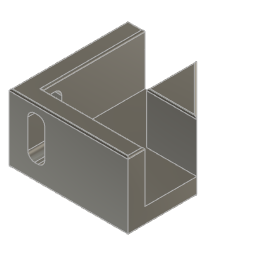
1515 (Autodesk Fusion 360 design; units mm, degrees)
Autodesk Fusion 360 part; units mm, degrees
sketch "Sketch1" plane through (0, 0, 0) normal (0, 0, 1) x (1, 0, 0)
  line L0 (0, 0) -> (35, 0)
  line L1 (35, 0) -> (35, 35)
  line L2 (35, 35) -> (0, 35)
  line L3 (0, 35) -> (0, 0)
  dimension "d1" = 35
  dimension "d2" = 35
  constraint horizontal L0
  constraint vertical L1
  constraint horizontal L2
  constraint vertical L3
  constraint coincident L0.start L3.end
  measures "d1" distance of L0.start L0.end
  measures "d2" distance of L0.start L2.end
extrude "Extrude1" add sketch "Sketch1" along normal blind 15
sketch "Sketch2" plane through (0, 0, 15) normal (0, 0, 1) x (-1, 0, 0)
  line L0 (0, -35) -> (0, 0)
  line L1 (0, 0) -> (-35, 0)
  line L2 (-35, 0) -> (-35, -35)
  line L3 (-35, -35) -> (0, -35)
  line L4 (0, -35) -> (-5, -35)
  line L5 (-5, -35) -> (-5, -35)
  line L6 (-5, -35) -> (0, -35)
  line L7 (0, -35) -> (0, -35)
  line L8 (-35, 0) -> (-35, -5)
  line L9 (-35, -5) -> (-5, -5)
  line L10 (0, -5) -> (0, 0)
  line L11 (0, 0) -> (-35, 0)
  line L12 (-35, 0) -> (-35, -5)
  line L13 (0, -35) -> (-5, -35)
  line L14 (-5, -35) -> (-5, -5)
  line L15 (-5, 0) -> (0, 0)
  line L16 (0, 0) -> (0, -35)
  line L17 (-5, -35) -> (-20.25, -35)
  line L18 (-35, -5) -> (-35, -20.25)
  line L19 (-5, -35) -> (-20.25, -35)
  line L20 (-20.25, -35) -> (-20.25, -20.25)
  line L21 (-20.25, -5) -> (-5, -5)
  line L22 (-5, -5) -> (-5, -35)
  line L23 (-35, -20.25) -> (-20.25, -20.25)
  line L24 (-5, -20.25) -> (-5, -5)
  line L25 (-5, -5) -> (-35, -5)
  line L26 (-35, -5) -> (-35, -20.25)
  line L27 (-20.25, -35) -> (-35, -20.25)
  dimension "d5" = 5
  dimension "d6" = 5
  dimension "d7" = 15.25
  dimension "d8" = 15.25
  constraint horizontal L4
  constraint horizontal L6
  constraint coincident L3 L4.end
  constraint coincident L0.start L3.end
  constraint coincident L1.end L2.start
  constraint coincident L2 L8.end
  constraint horizontal L9
  constraint vertical L10
  constraint horizontal L11
  constraint vertical L12
  constraint coincident L0.end L1.start
  constraint horizontal L13
  constraint vertical L14
  constraint horizontal L15
  constraint vertical L16
  constraint coincident L11 L15.start
  constraint coincident L3 L17.end
  constraint coincident L2 L18.end
  constraint horizontal L19
  constraint vertical L20
  constraint horizontal L21
  constraint vertical L22
  constraint coincident L9 L21.start
  constraint horizontal L23
  constraint vertical L24
  constraint horizontal L25
  constraint vertical L26
  measures "d5" distance of L0.start L4.end
  measures "d6" distance of L1.end L8.end
  measures "d7" distance of L4.end L17.end
  measures "d8" distance of L8.end L18.end
extrude "Extrude2" cut sketch "Sketch2" against normal blind 10 contours L2 L3 L9 L14 L17 L18 L19 L20 L21 L22 L23 L24 L25 L26 | L2 L3 L27
sketch "Sketch3" plane through (0, 0, 5) normal (0, 0, 1) x (-1, 0, 0)
  line L0 (-20.25, -35) -> (-35, -20.25)
  line L1 (-35, -20.25) -> (-35, -35)
  line L2 (-35, -35) -> (-20.25, -35)
extrude "Extrude3" cut sketch "Sketch3" against normal blind 5
sketch "Sketch4" plane through (0, 0, 15) normal (0, 0, 1) x (-1, 0, 0)
  line L0 (-5, -5) -> (-5, -35)
  line L1 (-5, -35) -> (0, -35)
  line L2 (0, -35) -> (0, 0)
  line L3 (0, 0) -> (-35, 0)
  line L4 (-35, 0) -> (-35, -5)
  line L5 (-35, -5) -> (-5, -5)
extrude "Extrude4" add sketch "Sketch4" 1 faces at (25.1667, 25.1667, 15) along normal blind 5
sketch "Sketch5" plane through (0, 0, 0) normal (-1, 0, 0) x (0, -1, 0)
  line L0 (-35, 0) -> (0, 0)
  line L1 (0, 0) -> (0, 20)
  line L2 (0, 20) -> (-35, 20)
  line L3 (-35, 20) -> (-35, 15)
  line L4 (-35, 15) -> (-35, 0)
  line L5 (0, 10) -> (-8, 10)
  circle A0 centre (-8, 10) radius 2.75
  dimension "d15" = 8
  dimension "d16" = 5.5
  constraint midpoint L1 L5.start
  constraint perpendicular L1 L5
  constraint coincident L5.end A0.centre
  measures "d15" distance of L5.start L5.end
  measures "d16" diameter of A0
extrude "Extrude5" cut sketch "Sketch5" against normal blind 6 contours A0
sketch "Sketch6" plane through (0, 0, 0) normal (0, -1, 0) x (1, 0, 0)
  line L0 (0, 0) -> (35, 0)
  line L1 (35, 0) -> (35, 20)
  line L2 (35, 20) -> (0, 20)
  line L3 (0, 20) -> (0, 0)
  line L4 (0, 10) -> (8, 10)
  circle A0 centre (8, 10) radius 2.75
  dimension "d19" = 8
  dimension "d20" = 5.5
  constraint midpoint L3 L4.start
  constraint perpendicular L3 L4
  constraint coincident L4.end A0.centre
  measures "d19" distance of L4.start L4.end
  measures "d20" diameter of A0
extrude "Extrude6" cut sketch "Sketch6" against normal blind 5 contours A0
sketch "Sketch7" plane through (0, 0, 0) normal (0, 0, -1) x (-1, 0, 0)
  line L0 (-19.3461, 18.8094) -> (-15.8812, 14.9126)
  line L1 (-9.8503, 21.6064) -> (-17.7571, 23.725)
  line L2 (-15.3958, 16.7239) -> (-18.8608, 20.6208)
  line L3 (-13.5199, 7.9115) -> (-7.7317, 13.6996)
  line L4 (-18.8608, 20.6208) -> (-18.3369, 22.576)
  line L5 (-14.8719, 18.6791) -> (-13.1329, 19.2291)
  line L6 (-21.4266, 10.0301) -> (-13.5199, 7.9115)
  line L7 (-12.4162, 11.0157) -> (-12.9264, 9.1115)
  line L8 (-7.7317, 13.6996) -> (-9.8503, 21.6064)
  line L9 (-17.7571, 23.725) -> (-23.5452, 17.9369)
  line L10 (-15.8812, 14.9126) -> (-15.3958, 16.7239)
  line L11 (-23.5452, 17.9369) -> (-21.4266, 10.0301)
  line L12 (-13.1329, 19.2291) -> (-14.6581, 13.5371)
  line L13 (-14.6581, 13.5371) -> (-12.4162, 11.0157)
  line L14 (-19.8564, 16.9052) -> (-19.3461, 18.8094)
  line L15 (-18.3369, 22.576) -> (-14.8719, 18.6791)
  line L16 (-12.9264, 9.1115) -> (-19.8564, 16.9052)
extrude "Extrude7" cut sketch "Sketch7" against normal blind 1
fillet "Fillet1" radius 0.25 1 faces at (15.8136, 13.1846, 0)
fillet "Fillet2" radius 0.25 1 faces at (18.2676, 11.6156, 1)
fillet "Fillet3" radius 0.5 1 faces at (30.4755, 10.0934, 0)
fillet "Fillet4" radius 0.5 2 faces at (25.1667, 25.1667, 20) (1.6667, 13.3333, 20)
hole "Hole1" at (27.7797, 27.4703, 10.5992) direction (-0.707107, -0.707107, 0) diameter 3 depth 2 tip angle 118
sketch "Sketch8" plane through (0, 0, 0) normal (0, -1, 0) x (1, 0, 0)
  circle A0 centre (8, 10) radius 2.75
  line L0 (35, 19.5) -> (0, 19.5)
  line L1 (0, 19.5) -> (0, 0.5)
  line L2 (0, 0.5) -> (35, 0.5)
  line L3 (35, 0.5) -> (35, 19.5)
extrude "Extrude8" add sketch "Sketch8" against normal blind 5 contours A0
sketch "Sketch9" plane through (0, 0, 0) normal (-1, 0, 0) x (0, -1, 0)
  circle A0 centre (-8, 10) radius 2.75
  line L0 (0, 19.5) -> (-35, 19.5)
  line L1 (-35, 19.5) -> (-35, 15)
  line L2 (-35, 15) -> (-35, 0.5)
  line L3 (-35, 0.5) -> (0, 0.5)
  line L4 (0, 0.5) -> (0, 19.5)
extrude "Extrude9" add sketch "Sketch9" against normal blind 5 contours A0
sketch "Sketch10" plane through (0, 0, 0) normal (0, -1, 0) x (1, 0, 0)
  line L0 (35, 19.5) -> (0, 19.5)
  line L1 (0, 19.5) -> (0, 0.5)
  line L2 (0, 0.5) -> (35, 0.5)
  line L3 (35, 0.5) -> (35, 19.5)
  line L4 (8.5, 17.5426) -> (7.5, 17.5426)
  line L5 (8.5, 5) -> (7.5, 5)
  line L6 (7.5, 17.5426) -> (8.5, 17.5426)
  line L7 (10.5, 15.5426) -> (10.5, 7)
  line L8 (8.5, 5) -> (7.5, 5)
  line L9 (5.5, 7) -> (5.5, 15.5426)
  arc A0 (7.5, 17.5426) -> (5.5, 15.5426) centre (7.5, 15.5426) ccw
  arc A1 (5.5, 7) -> (7.5, 5) centre (7.5, 7) ccw
  arc A2 (8.5, 5) -> (10.5, 7) centre (8.5, 7) ccw
  arc A3 (10.5, 15.5426) -> (8.5, 17.5426) centre (8.5, 15.5426) ccw
  dimension "d46" = 2
  constraint horizontal L4
  constraint horizontal L6
  constraint vertical L7
  constraint horizontal L8
  constraint vertical L9
  constraint tangent L6 A0
  constraint tangent L9 A0
  constraint tangent L9 A1
  constraint tangent L8 A1
  constraint equal A0 A1
  constraint tangent L7 A2
  constraint tangent L8 A2
  constraint equal A0 A2
  constraint tangent L7 A3
  constraint tangent L6 A3
  constraint equal A0 A3
  measures "d46" radius of A0
extrude "Extrude10" cut sketch "Sketch10" against normal blind 5 contours L4 L5 L6 L7 L8 L9 A0 A1 A2 A3
sketch "Sketch11" plane through (0, 0, 0) normal (-1, 0, 0) x (0, -1, 0)
  line L0 (0, 19.5) -> (-35, 19.5)
  line L1 (-35, 19.5) -> (-35, 15)
  line L2 (-35, 15) -> (-35, 0.5)
  line L3 (-35, 0.5) -> (0, 0.5)
  line L4 (0, 0.5) -> (0, 19.5)
  line L5 (-7.5, 17.5) -> (-8.5, 17.5)
  line L6 (-8.5, 5) -> (-7.5, 5)
  line L7 (-10.5, 15.5) -> (-10.5, 7)
  line L8 (-5.5, 7) -> (-5.5, 15.5)
  arc A0 (-8.5, 17.5) -> (-10.5, 15.5) centre (-8.5, 15.5) ccw
  arc A1 (-5.5, 15.5) -> (-7.5, 17.5) centre (-7.5, 15.5) ccw
  arc A2 (-7.5, 5) -> (-5.5, 7) centre (-7.5, 7) ccw
  arc A3 (-10.5, 7) -> (-8.5, 5) centre (-8.5, 7) ccw
  dimension "d52" = 2
  constraint perpendicular L6 L7
  constraint perpendicular L6 L8
  constraint tangent L7 A0
  constraint tangent L5 A0
  constraint tangent L5 A1
  constraint tangent L8 A1
  constraint equal A0 A1
  constraint tangent L8 A2
  constraint tangent L6 A2
  constraint equal A0 A2
  constraint tangent L6 A3
  constraint tangent L7 A3
  constraint equal A0 A3
  measures "d52" radius of A0
extrude "Extrude11" cut sketch "Sketch11" against normal blind 5 contours L5 L6 L7 L8 A0 A1 A2 A3
